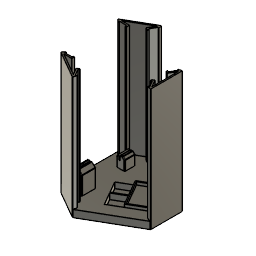
main-body-shell (Autodesk Fusion 360 design; units mm, degrees)
part number: 2026-07-17-13-50-10-986
Autodesk Fusion 360 part; units mm, degrees
note: some values were not read from the file. Chosen so that the rebuilt part matches the saved one: which pieces of a blend or face edit are solid.
sketch "Sketch2" plane through (0, 0, 0) normal (0, 0, 1) x (1, 0, 0)
  line L0 (0, 0) -> (58.9502, 0)
  line L1 (-48.6198, -39.9992) -> (-10.3305, -62.1056)
  line L2 (58.9502, 22.1063) -> (-10.3305, 62.1056)
  line L3 (-10.3305, 62.1056) -> (-48.6198, 39.9992)
  circle A0 centre (0, 0) radius 44.2127
  line L4 (-48.6198, -39.9992) -> (-48.6198, 39.9992)
  line L5 (58.9502, 22.1063) -> (58.9502, -22.1063)
  line L6 (0, 0) -> (-29.4751, -51.0524)
  line L7 (0, 0) -> (88.4253, 0) construction
  line L8 (0, 0) -> (88.4253, 0) construction
  line L9 (0, 0) -> (-29.4751, 51.0524)
  line L10 (-10.3305, -62.1056) -> (58.9502, -22.1063)
  dimension "d18" = 120
  dimension "d20" = 120
  dimension "d36" = 88.4253
  dimension "d37" = 62.1056
  dimension "d38" = 39.9992
  dimension "d39" = 22.1063
  dimension "d40" = 39.9992
  dimension "d41" = 29.4751
  constraint coincident L0.start A0.centre
  constraint horizontal L7
  constraint horizontal L8
  constraint coincident L0.end L7
  constraint midpoint L6.end L1
  constraint perpendicular L1 L6
  constraint midpoint L9.end L3
  constraint perpendicular L3 L9
  constraint midpoint L0.end L5
  constraint perpendicular L5 L8
  constraint parallel L1 L2
  constraint coincident L7.end L8.end
  constraint parallel L4 L5
  measures "d18" angle of L7 L9
  measures "d20" angle of L6 L8
  measures "d36" diameter of A0
  measures "d37" distance of L1.end L0
  measures "d38" distance of L1.start L0
  measures "d39" distance of L5.end L0
  measures "d40" distance of L3.end L0
  measures "d41" distance of L7.end L5
extrude "Extrude2" add sketch "Sketch2" along normal blind 10
sketch "Sketch3" plane through (0, 0, 10) normal (0, 0, 1) x (-1, 0, 0)
  line L0 (48.6198, 39.9992) -> (10.3305, 62.1056)
  line L1 (10.3305, 62.1056) -> (-58.9502, 22.1063)
  line L2 (-58.9502, 22.1063) -> (-58.9502, -22.1063)
  line L3 (-58.9502, -22.1063) -> (10.3305, -62.1056)
  line L4 (10.3305, -62.1056) -> (48.6198, -39.9992)
  line L5 (48.6198, -39.9992) -> (48.6198, 39.9992)
  line L6 (35, -38) -> (45, -38)
  line L7 (45, -38) -> (45, 38)
  line L8 (45, 38) -> (35, 38)
  line L9 (35, 38) -> (35, -38)
  line L10 (35, -38) -> (45, 38) construction
  line L11 (45, -38) -> (35, 38) construction
  line L12 (45, -38) -> (45, -36)
  line L13 (45, -36) -> (48.6198, -39.6198)
  line L14 (45, -36) -> (50.1191, -36) construction
  line L15 (45, 38) -> (45, 36)
  line L16 (45, 36) -> (48.6198, 39.6198)
  line L17 (45, 36) -> (50.1191, 36) construction
  line L18 (35, -36.2178) -> (33, -36.2178)
  line L19 (33, -36.2178) -> (33, -40.2178)
  line L20 (33, -40.2178) -> (48, -40.2178)
  line L21 (35, 0) -> (45, 0)
  line L22 (33, 36.2178) -> (33, 40.2178)
  line L23 (35, 36.2178) -> (33, 36.2178)
  line L24 (33, 40.2178) -> (48, 40.2178)
  line L25 (45, 36) -> (48.6198, 39.6198)
  line L26 (-53.6769, 20.9711) -> (-56.2365, 25.4044) construction
  line L27 (-48.8655, 12.202) -> (-47.8655, 10.4699)
  line L28 (13.8655, 48.4198) -> (14.8655, 46.6877)
  line L29 (10.409, 57.9711) -> (-55.409, 19.9711)
  line L30 (-53.6769, 20.9711) -> (-58.6216, 22.2961)
  line L31 (-55.409, 19.9711) -> (-53.6769, 20.9711)
  line L32 (15.409, 49.3109) -> (10.409, 57.9711)
  line L33 (18.3296, 48.6877) -> (10.8296, 61.6781)
  line L34 (15.409, 49.3109) -> (-55.409, 19.9711) construction
  line L35 (8.6769, 56.9711) -> (10.0018, 61.9158)
  line L36 (-51.3296, 8.4699) -> (-58.8296, 21.4603)
  line L37 (-55.409, 19.9711) -> (-50.409, 11.3109)
  line L38 (10.409, 57.9711) -> (8.6769, 56.9711)
  line L39 (-50.409, 11.3109) -> (15.409, 49.3109)
  line L40 (-47.8655, 10.4699) -> (-51.3296, 8.4699)
  line L41 (10.409, 57.9711) -> (-50.409, 11.3109) construction
  line L42 (-53.6769, 20.9711) -> (-58.6216, 22.2961)
  line L43 (14.8655, 46.6877) -> (18.3296, 48.6877)
  line L44 (8.6769, 56.9711) -> (6.1174, 61.4044) construction
  line L45 (-17.5, 30.3109) -> (-22.5, 38.9711)
  line L46 (10.3305, 62.1056) -> (-58.9502, 22.1063)
  line L47 (8.6769, -56.9711) -> (6.1174, -61.4044) construction
  line L48 (13.8655, -48.4198) -> (14.8655, -46.6877)
  line L49 (-48.8655, -12.202) -> (-47.8655, -10.4699)
  line L50 (-55.409, -19.9711) -> (10.409, -57.9711)
  line L51 (8.6769, -56.9711) -> (10.0018, -61.9158)
  line L52 (10.409, -57.9711) -> (8.6769, -56.9711)
  line L53 (-50.409, -11.3109) -> (-55.409, -19.9711)
  line L54 (-51.3296, -8.4699) -> (-58.8296, -21.4603)
  line L55 (-50.409, -11.3109) -> (10.409, -57.9711) construction
  line L56 (-53.6769, -20.9711) -> (-58.6216, -22.2961)
  line L57 (18.3296, -48.6877) -> (10.8296, -61.6781)
  line L58 (10.409, -57.9711) -> (15.409, -49.3109)
  line L59 (-55.409, -19.9711) -> (-53.6769, -20.9711)
  line L60 (15.409, -49.3109) -> (-50.409, -11.3109)
  line L61 (14.8655, -46.6877) -> (18.3296, -48.6877)
  line L62 (-55.409, -19.9711) -> (15.409, -49.3109) construction
  line L63 (8.6769, -56.9711) -> (10.0018, -61.9158)
  line L64 (-47.8655, -10.4699) -> (-51.3296, -8.4699)
  line L65 (-53.6769, -20.9711) -> (-56.2365, -25.4044) construction
  line L66 (-17.5, -30.3109) -> (-22.5, -38.9711)
  line L67 (-58.9502, -22.1063) -> (10.3305, -62.1056)
  line L68 (26.9416, -50.2057) -> (12.709, -58.4229)
  line L69 (26.9416, -50.2057) -> (44.2412, -40.2178)
  line L70 (28.4751, 49.3203) -> (12.709, 58.4229)
  line L71 (28.4751, 49.3203) -> (44.2412, 40.2178)
  line L72 (-56.9502, 0) -> (-56.9502, 18.2051)
  line L73 (-56.9502, 0) -> (-56.9502, -18.2051)
  point P0 (40, 0)
  point P1 (-20, 34.641)
  point P2 (-20, -34.641)
  dimension "d35" = 76
  dimension "d42" = 10
  dimension "d43" = 35
  dimension "d44" = 38
  dimension "d47" = 2
  dimension "d48" = 45
  dimension "d49" = 2
  dimension "d50" = 45
  dimension "d51" = 2
  dimension "d52" = 4
  dimension "d53" = 14.1115
  dimension "d54" = 106.9502
  dimension "d56" = 360
  dimension "d58" = 31.5322
  dimension "d59" = 18.2051
  dimension "d60" = 8.0584
  dimension "d63" = 91.9502
  dimension "d64" = 69.6593
  constraint horizontal L6
  constraint perpendicular L6 L7
  constraint parallel L6 L8
  constraint parallel L7 L9
  constraint coincident L10 P0
  constraint coincident L11 P0
  constraint perpendicular L6 L12
  constraint horizontal L14
  constraint coincident L5 L13.end
  constraint perpendicular L8 L15
  constraint horizontal L17
  constraint coincident L5 L16.end
  constraint coincident L9 L18.start
  constraint perpendicular L9 L18
  constraint perpendicular L18 L19
  constraint perpendicular L19 L20
  constraint equal L13 L14
  constraint equal L13 L17
  constraint midpoint L9 L21.start
  constraint midpoint L7 L21.end
  constraint symmetric L12.end L21 L15.end
  constraint symmetric L13.end L21 L16.end
  constraint symmetric L18.start L21 L23.start
  constraint symmetric L18.end L21 L22.start
  constraint symmetric L19.end L21 L22.end
  constraint symmetric L20.end L21 L24.end
  constraint coincident L57 L68.end
  constraint coincident L20 L69.end
  constraint parallel L68 L69
  constraint coincident L33 L70.end
  constraint coincident L24 L71.end
  constraint parallel L70 L71
  constraint vertical L68.end L70.end
  constraint vertical L69.end L71.end
  constraint equal L70 L71
  constraint coincident L36 L72.end
  constraint coincident L54 L73.end
  constraint horizontal origin L72.start
  constraint parallel L72 L73
  measures "d35" distance of L6.end L7.end
  measures "d42" distance of L7 L9
  measures "d43" distance of origin L9
  measures "d44" distance of origin L6
  measures "d47" distance of L6.end L12.end
  measures "d48" angle of L13 L14
  measures "d49" distance of L7.end L15.end
  measures "d50" angle of L16 L17
  measures "d51" distance of L18.start L18.end
  measures "d52" distance of L18.end L19.end
  measures "d53" distance of L2.end L18
  measures "d54" distance of L2 L20.end
  measures "d58" horizontal distance of L68.end L69.end
  measures "d59" vertical distance of L19.end L68.end
  measures "d60" horizontal distance of L6.start L68.start
  measures "d63" distance of L21.start L72
  measures "d64" distance of L68.end L72
extrude "Extrude3" add sketch "Sketch3" along normal blind 160 contours L0 L1 L5 L7 L8 L9 L15 L16 L22 L23 L24 L25 L28 L29 L32 L33 L35 L38 L39 L43 L46 L70 L71 | L3 L4 L5 L6 L7 L9 L12 L13 L18 L19 L20 L48 L50 L51 L52 L57 L58 L60 L61 L63 L67 L68 L69 | L1 L2 L3 L27 L29 L30 L31 L36 L37 L39 L40 L42 L46 L49 L50 L53 L54 L56 L59 L60 L64 L67 L72 L73
sketch "Sketch4" plane through (0, 0, 10) normal (0, 0, 1) x (-1, 0, 0)
  line L0 (45, -36) -> (48.6198, -39.6198)
  line L1 (48.6198, -39.6198) -> (48.6198, 39.6198)
  line L2 (48.6198, 39.6198) -> (45, 36)
  line L3 (45, 36) -> (45, 38)
  line L4 (45, 38) -> (35, 38)
  line L5 (35, 38) -> (35, 36.2178)
  line L6 (35, 36.2178) -> (33, 36.2178)
  line L7 (33, 36.2178) -> (33, 40.2178)
  line L8 (33, 40.2178) -> (44.2412, 40.2178)
  line L9 (44.2412, 40.2178) -> (12.709, 58.4229)
  line L10 (12.709, 58.4229) -> (18.3296, 48.6877)
  line L11 (18.3296, 48.6877) -> (14.8655, 46.6877)
  line L12 (14.8655, 46.6877) -> (13.8655, 48.4198)
  line L13 (13.8655, 48.4198) -> (15.409, 49.3109)
  line L14 (15.409, 49.3109) -> (10.409, 57.9711)
  line L15 (10.409, 57.9711) -> (8.6769, 56.9711)
  line L16 (8.6769, 56.9711) -> (10.0018, 61.9158)
  line L17 (10.0018, 61.9158) -> (-58.6216, 22.2961)
  line L18 (-58.6216, 22.2961) -> (-53.6769, 20.9711)
  line L19 (-53.6769, 20.9711) -> (-55.409, 19.9711)
  line L20 (-55.409, 19.9711) -> (-50.409, 11.3109)
  line L21 (-50.409, 11.3109) -> (-48.8655, 12.202)
  line L22 (-48.8655, 12.202) -> (-47.8655, 10.4699)
  line L23 (-47.8655, 10.4699) -> (-51.3296, 8.4699)
  line L24 (-51.3296, 8.4699) -> (-56.9502, 18.2051)
  line L25 (-56.9502, 18.2051) -> (-56.9502, -18.2051)
  line L26 (-56.9502, -18.2051) -> (-51.3296, -8.4699)
  line L27 (-51.3296, -8.4699) -> (-47.8655, -10.4699)
  line L28 (-47.8655, -10.4699) -> (-48.8655, -12.202)
  line L29 (-48.8655, -12.202) -> (-50.409, -11.3109)
  line L30 (-50.409, -11.3109) -> (-55.409, -19.9711)
  line L31 (-55.409, -19.9711) -> (-53.6769, -20.9711)
  line L32 (-53.6769, -20.9711) -> (-58.6216, -22.2961)
  line L33 (-58.6216, -22.2961) -> (10.0018, -61.9158)
  line L34 (10.0018, -61.9158) -> (8.6769, -56.9711)
  line L35 (8.6769, -56.9711) -> (10.409, -57.9711)
  line L36 (10.409, -57.9711) -> (15.409, -49.3109)
  line L37 (15.409, -49.3109) -> (13.8655, -48.4198)
  line L38 (13.8655, -48.4198) -> (14.8655, -46.6877)
  line L39 (14.8655, -46.6877) -> (18.3296, -48.6877)
  line L40 (18.3296, -48.6877) -> (12.709, -58.4229)
  line L41 (12.709, -58.4229) -> (44.2412, -40.2178)
  line L42 (44.2412, -40.2178) -> (33, -40.2178)
  line L43 (33, -40.2178) -> (33, -36.2178)
  line L44 (33, -36.2178) -> (35, -36.2178)
  line L45 (35, -36.2178) -> (35, -38)
  line L46 (35, -38) -> (45, -38)
  line L47 (45, -38) -> (45, -36)
  line L48 (24.5, 40) -> (26, 40)
  line L49 (24.5, 40) -> (26, -40.5) construction
  line L50 (26, 40) -> (24.5, -40.5) construction
  line L51 (24.5, 40) -> (19.5, 40)
  line L52 (19.5, 40) -> (19.5, 20)
  line L53 (19.5, 20) -> (24.5, 20)
  line L54 (24.5, 20) -> (24.5, 40)
  line L55 (26, 40) -> (31, 40)
  line L56 (31, 40) -> (31, 20)
  line L57 (31, 20) -> (26, 20)
  line L58 (26, 20) -> (26, 40)
  line L59 (31, 20) -> (19.5, 20)
  line L60 (19.5, 20) -> (19.5, 40)
  line L61 (19.5, 40) -> (31, 40)
  line L62 (31, 40) -> (31, 20)
  point P0 (25.25, -0.25)
  dimension "d67" = 1.5
  dimension "d75" = 5
  dimension "d76" = 20
  dimension "d77" = 5
  dimension "d121" = 2
  dimension "d122" = 78.1216
  dimension "d123" = 42.2961
  dimension "d124" = 83.8716
  dimension "d125" = 22.0461
  constraint horizontal L48
  constraint coincident L49 P0
  constraint coincident L50 P0
  constraint horizontal L51
  constraint vertical L52
  constraint horizontal L53
  constraint vertical L54
  constraint horizontal L55
  constraint vertical L56
  constraint horizontal L57
  constraint vertical L58
  constraint collinear L53 L57
  constraint horizontal L59
  constraint vertical L60
  constraint horizontal L61
  constraint vertical L62
  constraint equal L49 L50
  measures "d67" distance of L49.end L50.end
  measures "d75" distance of L48.start L51.end
  measures "d76" distance of L48.start L53.end
  measures "d77" distance of L48.end L55.end
  measures "d121" distance of L7 L56
  measures "d122" distance of L32.end L52
  measures "d123" distance of L32.end L53
  measures "d124" horizontal distance of L32.end P0
  measures "d125" vertical distance of L32.end P0
fillet "Fillet1" radius 1 6 edges at (-48.6198, -39.9992, 85) (-10.3305, -62.1056, 85) (-48.6198, 39.6198, 90) (-10.3305, 62.1056, 85) (58.6216, 22.2961, 90) (58.9502, -22.1063, 85)
sketch "Sketch5" plane through (0, 0, 10) normal (0, 0, 1) x (-1, 0, 0)
  arc A0 (-58.4502, 22.395) -> (-58.599, 22.29) centre (-57.9502, 21.529) ccw
  line L0 (-58.599, 22.29) -> (-53.6769, 20.9711)
  line L1 (-53.6769, 20.9711) -> (-55.409, 19.9711)
  line L2 (-55.409, 19.9711) -> (-50.409, 11.3109)
  line L3 (-50.409, 11.3109) -> (-48.8655, 12.202)
  line L4 (-48.8655, 12.202) -> (-47.8655, 10.4699)
  line L5 (-47.8655, 10.4699) -> (-51.3296, 8.4699)
  line L6 (-51.3296, 8.4699) -> (-56.9502, 18.2051)
  line L7 (-56.9502, 18.2051) -> (-56.9502, -18.2051)
  line L8 (-56.9502, -18.2051) -> (-51.3296, -8.4699)
  line L9 (-51.3296, -8.4699) -> (-47.8655, -10.4699)
  line L10 (-47.8655, -10.4699) -> (-48.8655, -12.202)
  line L11 (-48.8655, -12.202) -> (-50.409, -11.3109)
  line L12 (-50.409, -11.3109) -> (-55.409, -19.9711)
  line L13 (-55.409, -19.9711) -> (-53.6769, -20.9711)
  line L14 (-53.6769, -20.9711) -> (-58.2223, -22.1891)
  arc A1 (-58.9502, -22.1063) -> (-58.2223, -22.1891) centre (-58.4812, -21.2232) ccw
  line L15 (-58.9502, -22.1063) -> (9.8305, -61.8169)
  arc A2 (9.8305, -61.8169) -> (9.9958, -61.8932) centre (10.3305, -60.9509) ccw
  line L16 (9.9958, -61.8932) -> (8.6769, -56.9711)
  line L17 (8.6769, -56.9711) -> (10.409, -57.9711)
  line L18 (10.409, -57.9711) -> (15.409, -49.3109)
  line L19 (15.409, -49.3109) -> (13.8655, -48.4198)
  line L20 (13.8655, -48.4198) -> (14.8655, -46.6877)
  line L21 (14.8655, -46.6877) -> (18.3296, -48.6877)
  line L22 (18.3296, -48.6877) -> (12.709, -58.4229)
  line L23 (12.709, -58.4229) -> (44.2412, -40.2178)
  line L24 (44.2412, -40.2178) -> (33, -40.2178)
  line L25 (33, -40.2178) -> (33, -36.2178)
  line L26 (33, -36.2178) -> (35, -36.2178)
  line L27 (35, -36.2178) -> (35, -38)
  line L28 (35, -38) -> (45, -38)
  line L29 (45, -38) -> (45, -36)
  line L30 (45, -36) -> (48.3275, -39.3275)
  arc A3 (48.6198, -39.9992) -> (48.3275, -39.3275) centre (47.6204, -40.0346) ccw
  line L31 (48.6198, -39.9992) -> (48.6198, 39.4219)
  arc A4 (48.6198, 39.4219) -> (48.6032, 39.6032) centre (47.6198, 39.4219) ccw
  line L32 (48.6032, 39.6032) -> (45, 36)
  line L33 (45, 36) -> (45, 38)
  line L34 (45, 38) -> (35, 38)
  line L35 (35, 38) -> (35, 36.2178)
  line L36 (35, 36.2178) -> (33, 36.2178)
  line L37 (33, 36.2178) -> (33, 40.2178)
  line L38 (33, 40.2178) -> (44.2412, 40.2178)
  line L39 (44.2412, 40.2178) -> (12.709, 58.4229)
  line L40 (12.709, 58.4229) -> (18.3296, 48.6877)
  line L41 (18.3296, 48.6877) -> (14.8655, 46.6877)
  line L42 (14.8655, 46.6877) -> (13.8655, 48.4198)
  line L43 (13.8655, 48.4198) -> (15.409, 49.3109)
  line L44 (15.409, 49.3109) -> (10.409, 57.9711)
  line L45 (10.409, 57.9711) -> (8.6769, 56.9711)
  line L46 (8.6769, 56.9711) -> (9.9958, 61.8932)
  arc A5 (9.9958, 61.8932) -> (9.8305, 61.8169) centre (10.3305, 60.9509) ccw
  line L47 (9.8305, 61.8169) -> (-58.4502, 22.395)
  line L48 (-24.2002, 21.3846) -> (-4.9502, -11.9573)
  line L49 (-4.9502, -11.9573) -> (-23.31, -22.5573)
  line L50 (-23.31, -22.5573) -> (-42.56, 10.7846)
  line L51 (-42.56, 10.7846) -> (-24.2002, 21.3846)
  line L52 (-23.6512, 23.4337) -> (-2.9012, -12.5064)
  line L53 (-2.9012, -12.5064) -> (-23.859, -24.6064)
  line L54 (-23.859, -24.6064) -> (-44.609, 11.3337)
  line L55 (-44.609, 11.3337) -> (-23.6512, 23.4337)
  dimension "d82" = 38.5
  dimension "d83" = 21.2
  dimension "d84" = 18
  dimension "d85" = 54
  dimension "d87" = -1.5
  constraint perpendicular L48 L51
  constraint parallel L47 L51
  constraint perpendicular L49 L50
  constraint perpendicular L48 L49
  measures "d82" distance of L48.start L48.end
  measures "d83" distance of L48.start L50.end
  measures "d84" distance of L47 L51
  measures "d85" horizontal distance of A1.start L48.end
extrude "Extrude5" add sketch "Sketch5" along normal blind 4 contours L52 L53 L54 L55
sketch "Sketch6" plane through (0, 0, 10) normal (0, 0, 1) x (-1, 0, 0)
  arc A0 (-58.4502, 22.395) -> (-58.599, 22.29) centre (-57.9502, 21.529) ccw
  line L0 (-58.599, 22.29) -> (-53.6769, 20.9711)
  line L1 (-53.6769, 20.9711) -> (-55.409, 19.9711)
  line L2 (-55.409, 19.9711) -> (-50.409, 11.3109)
  line L3 (-50.409, 11.3109) -> (-48.8655, 12.202)
  line L4 (-48.8655, 12.202) -> (-47.8655, 10.4699)
  line L5 (-47.8655, 10.4699) -> (-51.3296, 8.4699)
  line L6 (-51.3296, 8.4699) -> (-56.9502, 18.2051)
  line L7 (-56.9502, 18.2051) -> (-56.9502, -18.2051)
  line L8 (-56.9502, -18.2051) -> (-51.3296, -8.4699)
  line L9 (-51.3296, -8.4699) -> (-47.8655, -10.4699)
  line L10 (-47.8655, -10.4699) -> (-48.8655, -12.202)
  line L11 (-48.8655, -12.202) -> (-50.409, -11.3109)
  line L12 (-50.409, -11.3109) -> (-55.409, -19.9711)
  line L13 (-55.409, -19.9711) -> (-53.6769, -20.9711)
  line L14 (-53.6769, -20.9711) -> (-58.2223, -22.1891)
  arc A1 (-58.9502, -22.1063) -> (-58.2223, -22.1891) centre (-58.4812, -21.2232) ccw
  line L15 (-58.9502, -22.1063) -> (9.8305, -61.8169)
  arc A2 (9.8305, -61.8169) -> (9.9958, -61.8932) centre (10.3305, -60.9509) ccw
  line L16 (9.9958, -61.8932) -> (8.6769, -56.9711)
  line L17 (8.6769, -56.9711) -> (10.409, -57.9711)
  line L18 (10.409, -57.9711) -> (15.409, -49.3109)
  line L19 (15.409, -49.3109) -> (13.8655, -48.4198)
  line L20 (13.8655, -48.4198) -> (14.8655, -46.6877)
  line L21 (14.8655, -46.6877) -> (18.3296, -48.6877)
  line L22 (18.3296, -48.6877) -> (12.709, -58.4229)
  line L23 (12.709, -58.4229) -> (44.2412, -40.2178)
  line L24 (44.2412, -40.2178) -> (33, -40.2178)
  line L25 (33, -40.2178) -> (33, -36.2178)
  line L26 (33, -36.2178) -> (35, -36.2178)
  line L27 (35, -36.2178) -> (35, -38)
  line L28 (35, -38) -> (45, -38)
  line L29 (45, -38) -> (45, -36)
  line L30 (45, -36) -> (48.3275, -39.3275)
  arc A3 (48.6198, -39.9992) -> (48.3275, -39.3275) centre (47.6204, -40.0346) ccw
  line L31 (48.6198, -39.9992) -> (48.6198, 39.4219)
  arc A4 (48.6198, 39.4219) -> (48.6032, 39.6032) centre (47.6198, 39.4219) ccw
  line L32 (48.6032, 39.6032) -> (45, 36)
  line L33 (45, 36) -> (45, 38)
  line L34 (45, 38) -> (35, 38)
  line L35 (35, 38) -> (35, 36.2178)
  line L36 (35, 36.2178) -> (33, 36.2178)
  line L37 (33, 36.2178) -> (33, 40.2178)
  line L38 (33, 40.2178) -> (44.2412, 40.2178)
  line L39 (44.2412, 40.2178) -> (12.709, 58.4229)
  line L40 (12.709, 58.4229) -> (18.3296, 48.6877)
  line L41 (18.3296, 48.6877) -> (14.8655, 46.6877)
  line L42 (14.8655, 46.6877) -> (13.8655, 48.4198)
  line L43 (13.8655, 48.4198) -> (15.409, 49.3109)
  line L44 (15.409, 49.3109) -> (10.409, 57.9711)
  line L45 (10.409, 57.9711) -> (8.6769, 56.9711)
  line L46 (8.6769, 56.9711) -> (9.9958, 61.8932)
  arc A5 (9.9958, 61.8932) -> (9.8305, 61.8169) centre (10.3305, 60.9509) ccw
  line L47 (9.8305, 61.8169) -> (-58.4502, 22.395)
  line L48 (-44.609, 11.3337) -> (-23.6512, 23.4337)
  line L49 (-23.6512, 23.4337) -> (-2.9012, -12.5064)
  line L50 (-2.9012, -12.5064) -> (-23.859, -24.6064)
  line L51 (-23.859, -24.6064) -> (-44.609, 11.3337)
  line L52 (-23.2182, 23.6837) -> (-5.8977, 33.6837)
  line L53 (-5.8977, 33.6837) -> (4.1023, 16.3632)
  line L54 (4.1023, 16.3632) -> (-13.2182, 6.3632)
  line L55 (-13.2182, 6.3632) -> (-23.2182, 23.6837)
  dimension "d90" = 20
  dimension "d91" = 20
  dimension "d92" = 16.5
  dimension "d93" = 0.5
  constraint parallel L47 L52
  constraint perpendicular L52 L53
  constraint perpendicular L53 L54
  measures "d90" distance of L52.start L52.end
  measures "d91" distance of L52.start L54.end
  measures "d92" distance of L47 L52
  measures "d93" distance of L49 L55
extrude "Extrude9" cut sketch "Sketch6" against normal blind 8 contours L52 L53 L54 L55
sketch "Sketch8" plane through (0, 0, 10) normal (0, 0, 1) x (-1, 0, 0)
  line L0 (13.8523, -0.5243) -> (-3.4682, -10.5243)
  line L1 (-3.4682, -10.5243) -> (-12.4682, 5.0641)
  line L2 (-12.4682, 5.0641) -> (4.8523, 15.0641)
  line L3 (4.8523, 15.0641) -> (13.8523, -0.5243)
  line L4 (4.1023, 16.3632) -> (-13.2182, 6.3632)
  line L5 (-23.6512, 23.4337) -> (-2.9012, -12.5064)
  dimension "d115" = 20
  dimension "d116" = 18
  dimension "d117" = 1.5
  dimension "d118" = 0.5
  constraint parallel L2 L4
  constraint perpendicular L0 L3
  constraint perpendicular L0 L1
  measures "d115" distance of L0.start L0.end
  measures "d116" distance of L0.start L2.end
  measures "d117" distance of L2 L4
  measures "d118" distance of L1 L5
extrude "Extrude10" cut sketch "Sketch8" against normal blind 8
sketch "Sketch9" plane through (0, 0, 10) normal (0, 0, 1) x (-1, 0, 0)
  line L0 (35, 36.2178) -> (33, 36.2178)
  line L1 (45, 38) -> (35, 38)
  line L2 (45, 36) -> (45, 38)
  line L3 (48.6198, 39.6198) -> (45, 36)
  line L4 (35, 38) -> (35, 36.2178)
  line L5 (19.5, 40) -> (19.5, 20)
  line L6 (24.5, 40) -> (26, 40)
  line L7 (31, 40) -> (31, 20)
  line L8 (26, 40) -> (31, 40)
  line L9 (19.5, 40) -> (31, 40)
  line L10 (14.8655, 46.6877) -> (13.8655, 48.4198)
  line L11 (13.8655, 48.4198) -> (15.409, 49.3109)
  line L12 (18.3296, 48.6877) -> (14.8655, 46.6877)
  line L13 (33, 40.2178) -> (44.2412, 40.2178)
  line L14 (33, 36.2178) -> (33, 40.2178)
  line L15 (19.5, 20) -> (24.5, 20)
  line L16 (24.5, 40) -> (19.5, 40)
  line L17 (31, 20) -> (19.5, 20)
  line L18 (31, 40) -> (31, 20)
  line L19 (26, 20) -> (26, 40)
  line L20 (31, 20) -> (26, 20)
  line L21 (19.5, 20) -> (19.5, 40)
  line L22 (24.5, 20) -> (24.5, 40)
  dimension "d126" = 5
  dimension "d127" = 20
  dimension "d128" = 5
  dimension "d129" = 2
  dimension "d130" = 19.5
  dimension "d131" = 40
  dimension "d132" = 4.6345
  dimension "d133" = 13.5
  dimension "d134" = 6.6877
  dimension "d135" = 0.2178
  dimension "d136" = 60
  dimension "d137" = 1.1704
  dimension "d138" = 5.6345
  dimension "d139" = 4.091
  dimension "d140" = 15.5
  dimension "d141" = 24.7412
  dimension "d142" = 25.5
  dimension "d143" = 29.1198
  dimension "d144" = 8.4198
  dimension "d145" = 9.3109
  dimension "d146" = 4
  dimension "d147" = 3.7822
  dimension "d148" = 2
  dimension "d149" = 0.3802
  constraint horizontal L6
  constraint horizontal L16
  constraint vertical L5
  constraint horizontal L15
  constraint vertical L22
  constraint horizontal L8
  constraint vertical L18
  constraint horizontal L20
  constraint vertical L19
  constraint collinear L15 L20
  constraint horizontal L17
  constraint vertical L21
  constraint horizontal L9
  constraint vertical L7
  measures "d126" distance of L6.start L5.start
  measures "d127" distance of L6.start L15.end
  measures "d128" distance of L6.end L7.start
  measures "d129" distance of L14 L18
  measures "d130" distance of origin L5
  measures "d131" distance of origin L9
  measures "d132" distance of L10.start L5
  measures "d133" distance of L5 L14
  measures "d134" distance of L10.start L9
  measures "d135" distance of L9 L13
  measures "d136" angle of L5 L12
  measures "d137" distance of L12.start L5
  measures "d138" distance of L10.end L5
  measures "d139" distance of L11.end L5
  measures "d140" distance of L4 L5
  measures "d141" distance of L13.end L5
  measures "d142" distance of L2 L5
  measures "d143" distance of L3.start L5
  measures "d144" distance of L10.end L8
  measures "d145" distance of L11.end L8
  measures "d146" distance of L2.start L8
  measures "d147" distance of L0 L8
  measures "d148" distance of L1 L8
  measures "d149" distance of L3.start L8
extrude "Extrude11" add sketch "Sketch9" along normal blind 10
sketch "Sketch10" plane through (0, 0, 20) normal (0, 0, 1) x (-1, 0, 0)
  line L0 (31, 40) -> (19.5, 40)
  line L1 (19.5, 40) -> (19.5, 20)
  line L2 (19.5, 20) -> (31, 20)
  line L3 (31, 20) -> (31, 40)
  line L4 (26, 20) -> (27.5, 20)
  line L5 (27.5, 20) -> (27.5, 40)
  line L6 (27.5, 40) -> (26, 40)
  line L7 (26, 40) -> (26, 20)
  line L8 (26, 20) -> (27.5, 40) construction
  line L9 (27.5, 20) -> (26, 40) construction
  point P0 (26.75, 30)
  dimension "d152" = 1.5
  dimension "d153" = 3.5
  constraint horizontal L4
  constraint perpendicular L4 L5
  constraint parallel L4 L6
  constraint parallel L5 L7
  constraint coincident L8 P0
  constraint coincident L9 P0
  constraint collinear L0 L6
  constraint collinear L2 L4
  measures "d152" distance of L5.end L6.end
  measures "d153" distance of L3 L5
extrude "Extrude12" add sketch "Sketch10" along normal blind 20 contours L0 L2 L3 L5 | L0 L1 L2 L7
chamfer "Chamfer1" distance 5 angle 45 1 edges at (-19.5, -30, 40)
fillet "Fillet2" radius 1 9 edges at (-19.5, -40, 22.5) (-19.5, -20, 22.5) (-19.5, -30, 35) (-22, -20, 37.5) (-22, -40, 37.5) (-24.5, -30, 40) (-26, -30, 40) (-25.25, -40, 40) (-25.25, -20, 40)
fillet "Fillet3" radius 1 4 edges at (-27.5, -30, 40) (-31, -30, 40) (-29.25, -20, 40) (-29.25, -40, 40)
fillet "Fillet4" radius 1 2 edges at (-31, -20, 24.5) (-30.7071, -20.2929, 39.7071)
sketch "Sketch11" plane through (0, 0, 10) normal (0, 0, 1) x (-1, 0, 0)
  line L0 (31, -20) -> (31, -35)
  line L1 (19.5, -20) -> (19.5, -35)
  line L2 (19.5, -20) -> (31, -20)
  line L3 (31, -35) -> (26, -35)
  line L4 (19.5, -35) -> (19.5, -20)
  line L5 (26, -35) -> (26, -20)
  line L6 (19.5, -35) -> (24.5, -35)
  line L7 (26, -20) -> (31, -20)
  line L8 (31, -35) -> (19.5, -35)
  line L9 (24.5, -20) -> (19.5, -20)
  line L10 (24.5, -20) -> (26, -20)
  line L11 (31, -20) -> (31, -35)
  line L12 (24.5, -35) -> (24.5, -20)
  line L13 (20.5, 20) -> (24.9142, 20)
  dimension "d164" = 5
  dimension "d165" = 15
  dimension "d166" = 5
  dimension "d167" = 55
  dimension "d168" = 19.5
  dimension "d169" = 11.5
  constraint horizontal L10
  constraint horizontal L9
  constraint vertical L1
  constraint horizontal L6
  constraint vertical L12
  constraint horizontal L7
  constraint vertical L0
  constraint horizontal L3
  constraint vertical L5
  constraint collinear L3 L6
  constraint horizontal L8
  constraint vertical L4
  constraint horizontal L2
  constraint vertical L11
  measures "d164" distance of L9.start L1.start
  measures "d165" distance of L9.start L6.end
  measures "d166" distance of L5.end L0.start
  measures "d167" distance of L8 L13
  measures "d168" distance of origin L1
  measures "d169" distance of L0 L1
extrude "Extrude13" add sketch "Sketch11" along normal blind 10
sketch "Sketch12" plane through (0, 0, 20) normal (0, 0, 1) x (-1, 0, 0)
  line L0 (31, -20) -> (19.5, -20)
  line L1 (19.5, -20) -> (19.5, -35)
  line L2 (19.5, -35) -> (31, -35)
  line L3 (31, -35) -> (31, -20)
  line L4 (19.5, -35) -> (19.5, -20)
  line L5 (27.5, -35) -> (27.5, -20)
  line L6 (31, -20) -> (31, -35)
  line L7 (26, -20) -> (19.5, -20)
  line L8 (19.5, -20) -> (31, -20)
  line L9 (19.5, -35) -> (26, -35)
  line L10 (31, -35) -> (19.5, -35)
  line L11 (19.5, -20) -> (19.5, -35)
  line L12 (26, -20) -> (27.5, -20)
  line L13 (27.5, -20) -> (31, -20)
  line L14 (26, -35) -> (26, -20)
  line L15 (31, -35) -> (27.5, -35)
  line L16 (31, -20) -> (31, -35)
  dimension "d172" = 6.5
  dimension "d173" = 15
  dimension "d174" = 3.5
  dimension "d175" = 11.5
  constraint horizontal L12
  constraint horizontal L7
  constraint vertical L11
  constraint horizontal L9
  constraint vertical L14
  constraint horizontal L13
  constraint vertical L16
  constraint horizontal L15
  constraint vertical L5
  constraint collinear L9 L15
  constraint horizontal L10
  constraint vertical L4
  constraint horizontal L8
  constraint vertical L6
  constraint collinear L0 L7
  constraint collinear L1 L4
  measures "d172" distance of L0.end L7.start
  measures "d173" distance of L9.end L7.start
  measures "d174" distance of L0.start L5.end
  measures "d175" distance of L11 L16
extrude "Extrude14" add sketch "Sketch12" along normal blind 6.5 contours L0 L2 L3 L5 L6 L8 L10 L13 L15 L16 | L0 L1 L2 L4 L7 L8 L9 L10 L11 L14
chamfer "Chamfer3" distance 3 angle 45 2 edges at (-19.5, 27.5, 26.5) (-31, 27.5, 26.5)
fillet "Fillet5" radius 1 18 edges at (-19.5, 27.5, 23.5) (-22.5, 27.5, 26.5) (-27.5, 27.5, 26.5) (-26, 27.5, 26.5) (-28, 27.5, 26.5) (-31, 27.5, 23.5) (-31, 20, 16.75) (-31, 35, 16.75) (-29.5, 20, 25) (-29.5, 35, 25) (-27.75, 20, 26.5) (-24.25, 20, 26.5) (-21, 20, 25) (-19.5, 20, 16.75) (-19.5, 35, 16.75) (-21, 35, 25) (-24.25, 35, 26.5) (-27.75, 35, 26.5)
